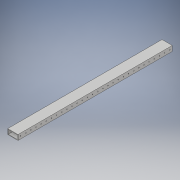
# Autodesk Inventor part: 30inVersaFrameUpright
Saved by Autodesk Inventor 2018.3 (Build 223284000, 284)
## iProperties
Created: 2019-09-02
Part Number: 30inVersaFrameUpright
Material: Generic
Document SubType Name: Modeling
Designer: Srinity
Density: 1 g/cm^3
Appearance: Default
Author: Srinity
Autodesk Inventor part; units mm, degrees
ref_plane "YZ Plane" through (0, 0, 0) normal (1, 0, 0) x (0, 1, 0)
ref_plane "XZ Plane" through (0, 0, 0) normal (0, 1, 0) x (-1, 0, 0)
ref_plane "XY Plane" through (0, 0, 0) normal (0, 0, 1) x (1, 0, 0)
sketch "Sketch1" plane through (0, 0, 0) normal (0, 0, 1) x (1, 0, 0)
  line L0 (24.1218, -9.7086) -> (-26.6782, -9.7086)
  line L1 (-26.6782, -9.7086) -> (-26.6782, 15.6914)
  line L2 (-26.6782, 15.6914) -> (24.1218, 15.6914)
  line L3 (24.1218, 15.6914) -> (24.1218, -9.7086)
  line L4 (21.5818, 13.1514) -> (-24.1382, 13.1514)
  line L5 (-24.1382, 13.1514) -> (-24.1382, -7.1686)
  line L6 (-24.1382, -7.1686) -> (21.5818, -7.1686)
  line L7 (21.5818, -7.1686) -> (21.5818, 13.1514)
  point P0 (0, 0)
  dimension "d0" = 25.4
  dimension "d1" = 50.8
  dimension "d2" = 2.54
  constraints: 16 end point, 4 parallel, 2 perpendicular, 1 horizontal, 3 other
  measures "d0" distance of L0.end L1.end
  measures "d1" distance of L1.end L2.end
  measures "d2" distance between parallel lines of L4 L2
extrude "Extrusion1" add sketch "Sketch1" along normal blind 762
sketch "Sketch2" plane through (24.1218, -9.7086, 0) normal (1, 0, 0) x (0, 0, -1)
  circle A0 centre (-12.7, 12.7) radius 2.0701
  line L0 (0, 25.4) -> (-762, 25.4) projected
  line L1 (0, 25.4) -> (0, 0) projected
  circle A1 centre (-38.1, 12.7) radius 2.0701
  circle A2 centre (-63.5, 12.7) radius 2.0701
  circle A3 centre (-88.9, 12.7) radius 2.0701
  circle A4 centre (-114.3, 12.7) radius 2.0701
  circle A5 centre (-139.7, 12.7) radius 2.0701
  circle A6 centre (-165.1, 12.7) radius 2.0701
  circle A7 centre (-190.5, 12.7) radius 2.0701
  circle A8 centre (-215.9, 12.7) radius 2.0701
  circle A9 centre (-241.3, 12.7) radius 2.0701
  circle A10 centre (-266.7, 12.7) radius 2.0701
  circle A11 centre (-292.1, 12.7) radius 2.0701
  circle A12 centre (-317.5, 12.7) radius 2.0701
  circle A13 centre (-342.9, 12.7) radius 2.0701
  circle A14 centre (-368.3, 12.7) radius 2.0701
  circle A15 centre (-393.7, 12.7) radius 2.0701
  circle A16 centre (-419.1, 12.7) radius 2.0701
  circle A17 centre (-444.5, 12.7) radius 2.0701
  circle A18 centre (-469.9, 12.7) radius 2.0701
  circle A19 centre (-495.3, 12.7) radius 2.0701
  circle A20 centre (-520.7, 12.7) radius 2.0701
  circle A21 centre (-546.1, 12.7) radius 2.0701
  circle A22 centre (-571.5, 12.7) radius 2.0701
  circle A23 centre (-596.9, 12.7) radius 2.0701
  circle A24 centre (-622.3, 12.7) radius 2.0701
  circle A25 centre (-647.7, 12.7) radius 2.0701
  circle A26 centre (-673.1, 12.7) radius 2.0701
  circle A27 centre (-698.5, 12.7) radius 2.0701
  circle A28 centre (-723.9, 12.7) radius 2.0701
  circle A29 centre (-749.3, 12.7) radius 2.0701
  point P0 (0, 9.7086)
  point P1 (0, 12.7)
  dimension "d5" = 12.7
  dimension "d6" = 4.1402
  dimension "d9" = 25.4
  constraints: 30 centre point, 1 horizontal, 1 horizontal alignment, 1 midpoint, 58 other
  measures "d5" distance from line of A0.centre L1
  measures "d6" diameter of A0
  measures "d9" distance of A0.centre A1.centre
extrude "Extrusion2" cut sketch "Sketch2" against normal through all
body "Solid1"
